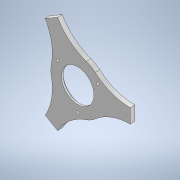
# Autodesk Inventor part: Tractor_Mobile
Saved by Autodesk Inventor 2022 (Build 260153070, 153G)
## iProperties
Created: 2022-03-05
Part Number: Tractor_Mobile
Material: Generic
Document SubType Name: Modeling
Designer: a laptop
Density: 1 g/cm^3
Appearance: Default
Author: a laptop
Autodesk Inventor part; units mm, degrees
ref_plane "YZ Plane" through (0, 0, 0) normal (1, 0, 0) x (0, 1, 0)
ref_plane "XZ Plane" through (0, 0, 0) normal (0, 1, 0) x (-1, 0, 0)
ref_plane "XY Plane" through (0, 0, 0) normal (0, 0, 1) x (1, 0, 0)
sketch "Sketch1" plane through (0, 0, 0) normal (0, 0, 1) x (1, 0, 0)
  circle A0 centre (0, 0) radius 55.075
  circle A1 centre (0, 0) radius 75.075
  circle A2 centre (0, -65.075) radius 4
  circle A3 centre (-56.3566, 32.5375) radius 4
  circle A4 centre (56.3566, 32.5375) radius 4
  line L0 (0, -65.075) -> (-56.3566, 32.5375) construction
  line L1 (-56.3566, 32.5375) -> (56.3566, 32.5375) construction
  line L2 (0, -65.075) -> (56.3566, 32.5375) construction
  line L3 (0, -61.075) -> (0, -55.075) construction
  line L4 (-52.8925, 30.5375) -> (-47.6963, 27.5375) construction
  line L5 (47.6963, 27.5375) -> (52.8925, 30.5375) construction
  dimension "d4" = 8
  dimension "d0" = 110.15
  dimension "d1" = 20
  dimension "d6" = 6
  constraints: 12 end point, 4 equal length, 3 line through centre, 3 point on circle, 2 centre point, 2 coincident, 2 vertical, 1 vertical alignment, 10 other
  measures "d0" diameter of A0
  measures "d1" radial gap between concentric circles of A0 A1
  measures "d6" distance of L3.start L3.end
extrude "Extrusion1" add sketch "Sketch1" along normal blind 8
sketch "Sketch2" plane through (0, 0, 8) normal (0, 0, 1) x (1, 0, 0)
  circle A0 centre (0, 0) radius 55.075 projected
  circle A1 centre (0, 0) radius 45.75
  circle A2 centre (0, 0) radius 75.075 projected
  circle A3 centre (56.3566, 32.5375) radius 4 projected
  circle A4 centre (-56.3566, 32.5375) radius 4 projected
  circle A5 centre (0, -65.075) radius 4 projected
  circle A6 centre (0, 0) radius 55.075 projected
  dimension "d7" = 91.5
  constraints: 1 centre point, 1 concentric
  measures "d7" diameter of A1
extrude "Extrusion2" add sketch "Sketch2" along normal blind 5 contours A0 | A2
sketch "Sketch3" plane through (0, 0, 13) normal (0, 0, 1) x (1, 0, 0)
  circle A0 centre (0, 0) radius 75.075 projected
  line L0 (72.362, 20) -> (147.404, 20)
  line L1 (147.404, 20) -> (147.404, -20)
  line L2 (147.404, -20) -> (72.362, -20)
  circle A1 centre (0, 0) radius 75.075 projected
  line L3 (-18.8605, -72.6673) -> (-56.3815, -137.6556)
  line L4 (-56.3815, -137.6556) -> (-91.0225, -117.6556)
  line L5 (-91.0225, -117.6556) -> (-53.5015, -52.6673)
  line L6 (-18.8605, 72.6673) -> (-56.3815, 137.6556)
  line L7 (-56.3815, 137.6556) -> (-91.0225, 117.6556)
  line L8 (-91.0225, 117.6556) -> (-53.5015, 52.6673)
  line L9 (147.404, 0) -> (-73.702, 127.6556) construction
  line L10 (-73.702, -127.6556) -> (-73.702, 127.6556) construction
  line L11 (147.404, 0) -> (-73.702, -127.6556) construction
  arc A2 (49.2286, 56.6816) -> (147.404, 20) centre (147.404, 169.7201) ccw
  arc A3 (147.404, -20) -> (49.2286, -56.6816) centre (147.404, -169.7201) ccw
  arc A4 (24.4734, -70.974) -> (-56.3815, -137.6556) centre (73.28, -212.5156) ccw
  arc A5 (-91.0225, -117.6556) -> (-73.702, -14.2925) centre (-220.6839, -42.7955) ccw
  arc A6 (-73.702, 14.2925) -> (-91.0225, 117.6556) centre (-220.6839, 42.7955) ccw
  arc A7 (-56.3815, 137.6556) -> (24.4734, 70.974) centre (73.28, 212.5156) ccw
  point P0 (24.4734, 70.974)
  point P1 (24.4734, -70.974)
  point P2 (-73.702, -14.2925)
  point P3 (49.2286, 56.6816)
  point P4 (49.2286, -56.6816)
  dimension "d10" = 40
  constraints: 24 end point, 14 point on circle, 9 equal length, 7 tangent, 6 centre point, 6 perpendicular, 6 point on line, 3 midpoint, 1 horizontal alignment, 11 other
  measures "d10" distance of L0.end L1.end
extrude "Extrusion3" add sketch "Sketch3" against normal up to surface (13 mm away) contours A0 L0 L1 L2 | A0 A2 L0 | L2 A3 A0 | A0 L6 A7 | A4 L3 A0 | A0 L8 L7 L6 | L3 L4 L5 A0 | A0 A6 L8 | L5 A5 A0
equation "\"d2\" = d4"
body "Solid1"
